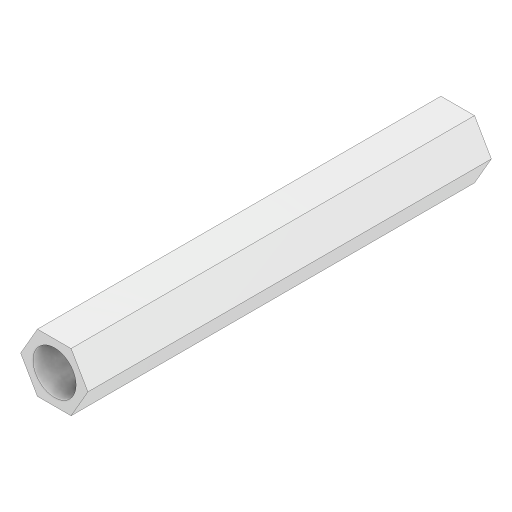
# Autodesk Inventor part: Supporter10
Saved by Autodesk Inventor 2023.2 (Build 272271000, 271)
## iProperties
Created: 2021-10-11
Part Number: Supporter10
Material: LCP 플라스틱
Document SubType Name: Modeling
Designer: BAEK
Density: 1.626 g/cm^3
Appearance: 매끄러움 - 흰색
Mass: 0.133259 g
Surface Area: 2.66922 cm^2
Volume: 0.081955 cm^3
Author: BAEK
Autodesk Inventor part; units mm, degrees
ref_plane "YZ Plane" through (0, 0, 0) normal (1, 0, 0) x (0, 1, 0)
ref_plane "XZ Plane" through (0, 0, 0) normal (0, 1, 0) x (-1, 0, 0)
ref_plane "XY Plane" through (0, 0, 0) normal (0, 0, 1) x (1, 0, 0)
sketch "스케치1" plane through (0, 0, 0) normal (0, 0, 1) x (1, 0, 0)
  circle A0 centre (0, 0) radius 1.6
  line L0 (-1.2705, 2.165) -> (1.2295, 2.165)
  line L1 (1.2295, 2.165) -> (4.1847, 2.165) construction
  line L2 (1.2295, 2.165) -> (2.4795, -0.0001)
  line L3 (1.2295, 2.165) -> (3.7295, 2.165) construction
  line L4 (2.4795, -0.0001) -> (1.2295, -2.1651)
  line L5 (1.2295, -2.1651) -> (-1.2705, -2.1651)
  line L6 (-1.2705, -2.1651) -> (-2.5205, -0.0001)
  line L7 (-2.5205, -0.0001) -> (-1.2705, 2.165)
  dimension "d0" = 3.2
  dimension "d2" = 2.5
  dimension "d3" = 2.5
  dimension "d4" = 60
  dimension "d5" = 2.5
  dimension "d6" = 2.165
  constraints: 16 end point, 4 horizontal, 2 parallel, 1 centre point, 1 coincident, 1 equal length
  measures "d0" diameter of A0
  measures "d2" distance of L0.start L0.end
  measures "d3" distance of L0.end L2.end
  measures "d4" angle of L2 L3
  measures "d5" distance of L2.end L4.end
  measures "d6" distance from line of L0 point (0, 0)
extrude "돌출1" add sketch "스케치1" along normal blind 30
